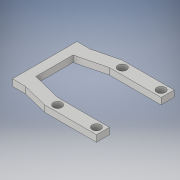
# Autodesk Inventor part: WheelSuspensionFork
Saved by Autodesk Inventor 2017 (Build 210142000, 142)
## iProperties
Created: 2018-05-09
Part Number: WheelSuspensionFork
Material: Generic
Document SubType Name: Modeling
Designer: User
Density: 1 g/cm^3
Appearance: Default
Author: User
Autodesk Inventor part; units mm, degrees
ref_plane "YZ Plane" through (0, 0, 0) normal (1, 0, 0) x (0, 1, 0)
ref_plane "XZ Plane" through (0, 0, 0) normal (0, 1, 0) x (-1, 0, 0)
ref_plane "XY Plane" through (0, 0, 0) normal (0, 0, 1) x (1, 0, 0)
sketch "Sketch1" plane through (0, 0, 0) normal (0, 1, 0) x (-1, 0, 0)
  line L0 (0, 0) -> (88.9, 0)
  line L1 (88.9, 0) -> (88.9, -76.2)
  line L2 (88.9, -76.2) -> (0, -76.2)
  line L3 (0, -76.2) -> (0, 0)
  line L4 (79.375, -19.8437) -> (79.375, -56.3563)
  line L5 (76.2, -69.85) -> (88.9, -69.85)
  line L6 (88.9, -69.85) -> (88.9, -6.35)
  line L7 (0, -12.7) -> (50.8, -12.7)
  line L8 (0, -63.5) -> (50.8, -63.5)
  line L9 (50.8, -63.5) -> (79.375, -56.3563)
  line L10 (50.8, -76.2) -> (76.2, -69.85)
  line L11 (50.8, -12.7) -> (79.375, -19.8437)
  line L12 (50.8, 0) -> (76.2, -6.35)
  line L13 (76.2, -6.35) -> (88.9, -6.35)
  dimension "d0" = 88.9
  dimension "d1" = 76.2
  dimension "d2" = 12.7
  dimension "d4" = 6.35
  dimension "d5" = 50.8
  dimension "d6" = 12.7
  dimension "d7" = 50.8
  dimension "d8" = 50.8
  dimension "d9" = 12.7
  dimension "d10" = 50.8
  dimension "d15" = 12.7
  dimension "d16" = 6.35
  dimension "d17" = 9.525
  constraints: 28 end point, 6 point on line, 5 parallel, 3 perpendicular, 2 horizontal, 1 collinear
  measures "d0" distance of L1.end L2.end
  measures "d1" distance of L0.end L1.end
  measures "d2" distance of L5.end L5.start
  measures "d4" distance between parallel lines of L2 L5
  measures "d5" distance of L7.start L7.end
  measures "d6" distance between parallel lines of L0 L7
  measures "d7" distance of L0.start L12.start
  measures "d8" distance of L8.start L8.end
  measures "d9" distance between parallel lines of L2 L8
  measures "d10" distance from line of L3 L10.start
  measures "d15" distance from line of L1 L12.end
  measures "d16" distance between parallel lines of L0 L13
  measures "d17" distance between parallel lines of L6 L4
extrude "Extrusion1" add sketch "Sketch1" along normal blind 6.35 contours L0 L12 L13 L1 L5 L10 L2 L3 L8 L9 L4 L11 L7
sketch "Sketch2" plane through (0, 6.35, 0) normal (0, 1, 0) x (1, 0, 0)
  line L0 (0, 0) -> (0, 12.7) projected
  line L1 (0, 12.7) -> (-50.8, 12.7) projected
  line L2 (-50.8, 12.7) -> (-79.375, 19.8437) projected
  line L3 (-79.375, 19.8437) -> (-79.375, 56.3563) projected
  line L4 (-79.375, 56.3563) -> (-50.8, 63.5) projected
  line L5 (-50.8, 63.5) -> (0, 63.5) projected
  line L6 (0, 63.5) -> (0, 76.2) projected
  line L7 (0, 76.2) -> (-50.8, 76.2) projected
  line L8 (-50.8, 76.2) -> (-76.2, 69.85) projected
  line L9 (-76.2, 69.85) -> (-88.9, 69.85) projected
  line L10 (-88.9, 69.85) -> (-88.9, 6.35) projected
  line L11 (-88.9, 6.35) -> (-76.2, 6.35) projected
  line L12 (-76.2, 6.35) -> (-50.8, 0) projected
  line L13 (-50.8, 0) -> (0, 0) projected
  point P0 (-6.35, 6.35)
  point P1 (-6.35, 69.85)
  dimension "d25" = 12.7
  dimension "d26" = 50.8
  dimension "d27" = 6.35
  dimension "d28" = 6.35
  dimension "d29" = 6.35
  dimension "d30" = 6.35
  measures "d25" distance of L0.start L0.end
  measures "d26" distance of L12.end L0.start
  measures "d27" distance from line of L13 point (-6.35, 6.35)
  measures "d28" distance from line of L0 point (-6.35, 6.35)
  measures "d29" distance from line of L6 point (-6.35, 69.85)
  measures "d30" distance from line of L7 point (-6.35, 69.85)
hole "Hole1" at (-6.35, 6.35, -6.35) at (-6.35, 6.35, -69.85) direction (0, -1, 0) diameter 8.4582 depth 19.05 tip angle 118
sketch "Sketch3" plane through (0, 6.35, 0) normal (0, 1, 0) x (1, 0, 0)
  circle A0 centre (-6.35, 6.35) radius 4.2291 projected
  circle A1 centre (-6.35, 69.85) radius 4.2291 projected
  line L0 (0, 0) -> (0, 12.7) projected
  line L1 (0, 12.7) -> (-50.8, 12.7) projected
  line L2 (-50.8, 12.7) -> (-79.375, 19.8437) projected
  line L3 (-79.375, 19.8437) -> (-79.375, 56.3563) projected
  line L4 (-79.375, 56.3563) -> (-50.8, 63.5) projected
  line L5 (-50.8, 63.5) -> (0, 63.5) projected
  line L6 (0, 63.5) -> (0, 76.2) projected
  line L7 (0, 76.2) -> (-50.8, 76.2) projected
  line L8 (-50.8, 76.2) -> (-76.2, 69.85) projected
  line L9 (-76.2, 69.85) -> (-88.9, 69.85) projected
  line L10 (-88.9, 69.85) -> (-88.9, 6.35) projected
  line L11 (-88.9, 6.35) -> (-76.2, 6.35) projected
  line L12 (-76.2, 6.35) -> (-50.8, 0) projected
  line L13 (-50.8, 0) -> (0, 0) projected
  point P0 (-44.45, 6.35)
  point P1 (-44.45, 69.85)
  dimension "d31" = 38.1
  dimension "d32" = 38.1
  dimension "d33" = 6.35
  dimension "d34" = 6.35
  dimension "d35" = 6.35
  measures "d31" distance of point (-44.45, 6.35) A0.centre
  measures "d32" distance of A1.centre point (-44.45, 69.85)
  measures "d33" distance from line of L7 point (-44.45, 69.85)
  measures "d34" distance from line of L7 A1.centre
  measures "d35" distance from line of L13 point (-44.45, 6.35)
hole "Hole2" at (-44.45, 6.35, -6.35) at (-44.45, 6.35, -69.85) direction (0, -1, 0) diameter 8.4582 depth 19.05 tip angle 118
equation "\"d2\" = d15"
equation "\"d4\" = d3"
equation "\"d5\" = d10"
equation "\"d7\" = d5"
equation "\"d8\" = d10"
equation "\"d9\" = d6"
equation "\"d27\" = 0.5 * d25"
equation "\"d28\" = d30"
equation "\"d29\" = d28"
equation "\"d30\" = d27"
equation "\"d33\" = d34"
equation "\"d35\" = d34"
equation "\"d3\" = 6.35"
body "Solid1"
